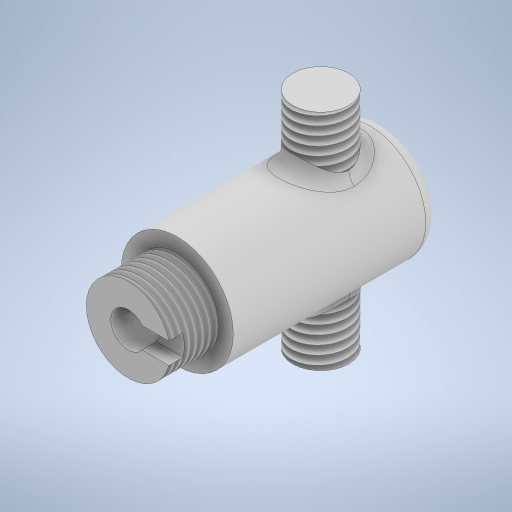
# Autodesk Inventor part: HUDSON-1-42
Saved by Autodesk Inventor 2024.2 (Build 282272000, 272)
## iProperties
Created: 2024-10-10
Part Number: HUDSON-1-42
Material: Generic
Document SubType Name: Modeling
Designer: Precisión-05
Density: 1 g/cm^3
Appearance: Default
Author: Precisión-05
Autodesk Inventor part; units mm, degrees
sketch "Sketch1" plane through (0, 0, 0) normal (0, 1, 0) x (-1, 0, 0)
  circle A0 centre (0, 0) radius 8
  dimension "d0" = 16
  constraints: 1 centre point, 1 coincident
  measures "d0" diameter of A0
extrude "Extrusion1" add sketch "Sketch1" along normal blind 29.5
sketch "Sketch2" plane through (0, 0, 0) normal (0, -1, 0) x (1, 0, 0)
  point P0 (0, 0)
  point P1 (0, 0)
  constraints: 1 coincident
sketch "Sketch3" plane through (0, 0, 0) normal (0, -1, 0) x (1, 0, 0)
  circle A0 centre (0, 0) radius 8 projected
  circle A1 centre (0, 0) radius 6
  circle A2 centre (0, 0) radius 8
  dimension "d10" = 12
  dimension "d11" = 16
  constraints: 2 centre point, 2 coincident
  measures "d10" diameter of A1
  measures "d11" diameter of A2
extrude "Extrusion2" add sketch "Sketch3" along normal blind 7 contours A1
thread "Thread1" size "M12x1" class "6g" standard "ANSI Metric M Profile" full length
sketch "Sketch4" plane through (0, -7, 0) normal (0, -1, 0) x (1, 0, 0)
  point P0 (0, 0)
  point P1 (0, 0)
  constraints: 1 coincident
hole "Hole2" at (0, -7, 0) direction (0, 1, 0) diameter 5 depth 32
ref_plane "Work Plane1" through (0, 0, 8) normal (0, 0, 1) x (1, 0, 0)
sketch "Sketch6" plane through (0, 0, 8) normal (0, 0, 1) x (1, 0, 0)
  line L0 (8, 29.5) -> (-8, 29.5) projected
  line L1 (8, 0) -> (-8, 0) projected
  line L2 (-8, 29.5) -> (8, 29.5)
  line L3 (8, 29.5) -> (8, 0)
  line L4 (8, 0) -> (-8, 0)
  line L5 (-8, 0) -> (-8, 29.5)
  line L6 (0, 29.5) -> (0, 20.5)
  circle A0 centre (0, 20.5) radius 4
  point P0 (0, 0)
  dimension "d28" = 9
  dimension "d29" = 8
  constraints: 10 end point, 2 parallel, 1 centre point, 1 coincident, 1 horizontal, 1 midpoint, 1 perpendicular, 1 vertical
  measures "d28" distance of L6.start L6.end
  measures "d29" diameter of A0
extrude "Extrusion4" add sketch "Sketch6" along normal blind 8 and the other way blind 3.5 contours A0
ref_plane "Work Plane2" through (0, 0, -8) normal (0, 0, 1) x (1, 0, 0)
sketch "Sketch7" plane through (0, 0, -8) normal (0, 0, 1) x (1, 0, 0)
  spline S0 degree 5 poles (4, 20.5) (3.9993, 21.7578) (3.5081, 23.0176) (2.5099, 24.0117) (-0.0068, 24.9921) (-2.5209, 24.0036) (-3.5135, 23.0068) (-4.4912, 20.4912) (-3.5035, 17.9797) (-2.5076, 16.9872) (0.0066, 16.0092) (2.5165, 16.9948) (3.5103, 17.988) (3.9993, 19.2449) (4, 20.5) knots 0 0 0 0 0 0 0.250295 0.250295 0.250295 0.500334 0.500334 0.500334 0.750253 0.750253 0.750253 1 1 1 1 1 1 projected
  line L0 (8, 29.5) -> (-8, 29.5) projected
  line L1 (8, 0) -> (-8, 0) projected
  line L2 (8, 0) -> (-8, 0) projected
  line L3 (-8, 29.5) -> (8, 29.5)
  line L4 (8, 29.5) -> (8, 0)
  line L5 (8, 0) -> (-8, 0)
  line L6 (-8, 0) -> (-8, 29.5)
  circle A0 centre (0, 20.5) radius 4
  point P0 (0, 0)
  constraints: 8 end point, 2 parallel, 1 centre point, 1 horizontal, 1 perpendicular, 1 other
extrude "Extrusion5" add sketch "Sketch7" along normal blind 3.5 and the other way blind 8 contours S0
thread "Thread2" size "M8x1.25" class "6g" standard "ANSI Metric M Profile" full length
fillet "Fillet1" radius 2 6 edges at (3.039, 23.1008, -7.4003) (-3.9999, 20.5, -6.9283) (3.0391, 17.8993, -7.4003) (3.0331, 17.8923, 7.4027) (-4, 20.4966, 6.9282) (3.0331, 23.1077, 7.4027)
fillet "Fillet2" radius 2 1 edges at (8, 29.5, 0)
ref_plane "Work Plane3" through (6, 0, 0) normal (1, 0, 0) x (0, 1, 0)
sketch "Sketch8" plane through (6, 0, 0) normal (1, 0, 0) x (0, 1, 0)
  line L0 (-7, 6) -> (-7, -6) projected
  line L1 (0, -6) -> (0, 6) projected
  line L2 (0, -6) -> (0, 6) projected
  line L3 (0, 6) -> (-7, 6)
  line L4 (-7, 6) -> (-7, -6)
  line L5 (-7, -6) -> (0, -6)
  line L6 (0, -6) -> (0, 6)
  line L7 (-9, 1.5) -> (-5, 1.5)
  line L8 (-5, 1.5) -> (-5, -1.5)
  line L9 (-5, -1.5) -> (-9, -1.5)
  line L10 (-9, -1.5) -> (-9, 1.5)
  line L11 (-9, 1.5) -> (-5, -1.5) construction
  line L12 (-5, 1.5) -> (-9, -1.5) construction
  point P0 (0, 0)
  point P1 (-7, 0)
  point P2 (-7, 1.5)
  point P3 (-7, -1.5)
  dimension "d44" = 4
  dimension "d45" = 3
  constraints: 20 end point, 4 parallel, 3 midpoint, 2 horizontal, 2 perpendicular
  measures "d44" distance of L8.end L9.end
  measures "d45" distance of L7.end L8.end
extrude "Extrusion6" cut sketch "Sketch8" against normal blind 4 contours L7 L8 L9 L0
body "Solid1"
